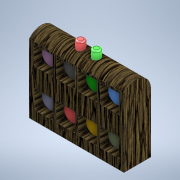
# Autodesk Inventor part: TreasureChestFinal
Saved by Autodesk Inventor 2021 (Build 250183000, 183)
## iProperties
Created: 2021-03-02
Part Number: TreasureChestFinal
Material: Generic
Document SubType Name: Modeling
Designer: con_c_000
Density: 1 g/cm^3
Appearance: Default
Author: con_c_000
Autodesk Inventor part; units mm, degrees
ref_plane "YZ Plane" through (0, 0, 0) normal (1, 0, 0) x (0, 1, 0)
ref_plane "XZ Plane" through (0, 0, 0) normal (0, 1, 0) x (-1, 0, 0)
ref_plane "XY Plane" through (0, 0, 0) normal (0, 0, 1) x (1, 0, 0)
sketch "Sketch1" plane through (0, 0, 0) normal (0, 1, 0) x (-1, 0, 0)
  line L0 (923.5659, 4.2179) -> (-600.4341, 4.2179)
  line L1 (-600.4341, 4.2179) -> (-600.4341, -300.5821)
  line L2 (-600.4341, -300.5821) -> (923.5659, -300.5821)
  line L3 (923.5659, -300.5821) -> (923.5659, 4.2179)
  point P0 (0, 0)
  dimension "d0" = 1524
  dimension "d1" = 304.8
  constraints: 8 end point, 2 parallel, 1 horizontal, 1 perpendicular
  measures "d0" distance of L2.end L1.end
  measures "d1" distance of L1.end L0.end
extrude "Extrusion1" add sketch "Sketch1" along normal blind 1219.2
sketch "Sketch2" plane through (-923.5659, 0, 4.2179) normal (0, 0, 1) x (1, 0, 0)
  circle A0 centre (228.6, 304.8) radius 127
  circle A1 centre (584.2, 304.8) radius 127
  circle A2 centre (939.8, 304.8) radius 127
  circle A3 centre (1295.4, 304.8) radius 127
  circle A4 centre (1295.4, 914.4) radius 127
  circle A5 centre (939.8, 914.4) radius 127
  circle A6 centre (584.2, 914.4) radius 127
  circle A7 centre (228.6, 914.4) radius 127
  line L0 (1524, 0) -> (1524, 1219.2) projected
  line L1 (0, 0) -> (0, 1219.2) projected
  line L2 (0, 1219.2) -> (1524, 1219.2) projected
  point P0 (923.5659, 0)
  dimension "d11" = 254
  dimension "d19" = 355.6
  dimension "d20" = 355.6
  dimension "d21" = 304.8
  dimension "d22" = 609.6
  dimension "d23" = 355.6
  dimension "d24" = 228.6
  constraints: 8 centre point, 7 equal radius, 6 horizontal alignment, 4 vertical alignment
  measures "d11" diameter of A7
  measures "d19" distance of A6.centre A5.centre
  measures "d20" distance of A4.centre A5.centre
  measures "d21" distance from line of L2 A7.centre
  measures "d22" distance of A0.centre A7.centre
  measures "d23" distance of A6.centre A7.centre
  measures "d24" distance from line of L1 A7.centre
extrude "Extrusion2" add sketch "Sketch2" along normal blind 25.4
sketch "Sketch3" plane through (-923.5659, 0, 4.2179) normal (0, 0, 1) x (1, 0, 0)
  line L0 (0, 1219.2) -> (1524, 1219.2) projected
  line L1 (0, 1219.2) -> (1524, 1219.2)
  line L2 (1524, 1219.2) -> (1524, 0)
  line L3 (1524, 0) -> (0, 0)
  line L4 (0, 0) -> (0, 1219.2)
  line L5 (76.2, 1066.8) -> (381, 1066.8)
  line L6 (381, 1066.8) -> (381, 762)
  line L7 (381, 762) -> (76.2, 762)
  line L8 (76.2, 762) -> (76.2, 1066.8)
  line L9 (431.8, 762) -> (736.6, 762)
  line L10 (736.6, 762) -> (736.6, 1066.8)
  line L11 (736.6, 1066.8) -> (431.8, 1066.8)
  line L12 (431.8, 1066.8) -> (431.8, 762)
  line L13 (787.4, 1066.8) -> (1092.2, 1066.8)
  line L14 (1092.2, 1066.8) -> (1092.2, 762)
  line L15 (1092.2, 762) -> (787.4, 762)
  line L16 (787.4, 762) -> (787.4, 1066.8)
  line L17 (1143, 762) -> (1447.8, 762)
  line L18 (1447.8, 762) -> (1447.8, 1066.8)
  line L19 (1447.8, 1066.8) -> (1143, 1066.8)
  line L20 (1143, 1066.8) -> (1143, 762)
  line L21 (84.918, 457.2) -> (381, 457.2)
  line L22 (381, 457.2) -> (381, 152.4)
  line L23 (381, 152.4) -> (84.918, 152.4)
  line L24 (84.918, 152.4) -> (84.918, 457.2)
  line L25 (431.8, 152.4) -> (736.6, 152.4)
  line L26 (736.6, 152.4) -> (736.6, 457.2)
  line L27 (736.6, 457.2) -> (431.8, 457.2)
  line L28 (431.8, 457.2) -> (431.8, 152.4)
  line L29 (787.4, 457.2) -> (1092.2, 457.2)
  line L30 (1092.2, 457.2) -> (1092.2, 152.4)
  line L31 (1092.2, 152.4) -> (787.4, 152.4)
  line L32 (787.4, 152.4) -> (787.4, 457.2)
  line L33 (1143, 152.4) -> (1447.8, 152.4)
  line L34 (1447.8, 152.4) -> (1447.8, 457.2)
  line L35 (1447.8, 457.2) -> (1143, 457.2)
  line L36 (1143, 457.2) -> (1143, 152.4)
  point P0 (923.5659, 0)
  point P1 (1524, 1219.2)
  dimension "d25" = 304.8
  dimension "d26" = 304.8
  dimension "d27" = 152.4
  dimension "d28" = 50.8
  dimension "d29" = 76.2
  dimension "d30" = 50.8
  dimension "d31" = 50.8
  dimension "d32" = 0
  dimension "d33" = 0
  dimension "d34" = 0
  dimension "d35" = 304.8
  dimension "d36" = 304.8
  dimension "d37" = 0
  constraints: 72 end point, 17 parallel, 13 point on line, 10 horizontal, 9 perpendicular, 5 equal length
  measures "d25" distance of L5.start L5.end
  measures "d26" distance of L7.end L5.start
  measures "d27" distance between parallel lines of L0 L5
  measures "d28" distance between parallel lines of L6 L12
  measures "d29" distance between parallel lines of L4 L8
  measures "d30" distance between parallel lines of L16 L10
  measures "d31" distance between parallel lines of L20 L14
  measures "d32" distance between parallel lines of L13 L19
  measures "d33" distance between parallel lines of L34 L18
  measures "d34" distance between parallel lines of L27 L21
  measures "d35" distance of L23.end L21.start
  measures "d36" distance between parallel lines of L7 L21
  measures "d37" distance between parallel lines of L25 L31
extrude "Extrusion3" add sketch "Sketch3" along normal blind 127
sketch "Sketch5" plane through (0, 1219.2, 0) normal (0, 1, 0) x (1, 0, 0)
  line L0 (600.4341, 300.5821) -> (600.4341, -131.2179) projected
  line L1 (600.4341, 300.5821) -> (-923.5659, 300.5821) projected
  line L2 (-923.5659, 300.5821) -> (-923.5659, -131.2179) projected
  line L3 (600.4341, -131.2179) -> (-923.5659, -131.2179) projected
  point P0 (0, 0)
extrude "Extrusion4" add sketch "Sketch5" along normal blind 254
sketch "Sketch6" plane through (-923.5659, 0, -300.5821) normal (-1, 0, 0) x (0, 0, 1)
  line L0 (431.8, 0) -> (431.8, 1473.2) projected
  line L1 (0, 0) -> (0, 1473.2) projected
  arc A0 (431.8, 1102.0767) -> (0, 944.9143) centre (239.7521, 957.9625) ccw
  line L2 (431.8, 1102.0767) -> (0, 944.9143) construction
  line L3 (431.8, 1102.0767) -> (891.312, 1102.0767) construction
  line L4 (0, 944.9143) -> (431.8, 944.9143)
  line L5 (431.8, 944.9143) -> (431.8, 1473.2)
  line L6 (431.8, 1473.2) -> (0, 1473.2)
  line L7 (0, 1473.2) -> (0, 944.9143)
  point P0 (300.5821, 0)
  point P1 (0, 971.0107)
  dimension "d42" = 160
  constraints: 12 end point, 2 horizontal, 2 parallel, 2 point on circle, 2 point on line, 1 centre point, 1 equal length, 1 perpendicular
  measures "d42" angle of L2 L3
extrude "Extrusion5" cut sketch "Sketch6" against normal through all contours A0 L1 L6 L0
ref_plane "Work Plane1" through (-923.5659, 1198.0694, -60.83) normal (0, -1, 0) x (1, 0, 0)
sketch "Sketch7" plane through (-923.5659, 1198.0694, -60.83) normal (0, -1, 0) x (1, 0, 0)
  circle A0 centre (635, 0.1041) radius 63.5
  circle A1 centre (889, 0.1041) radius 63.5
  line L0 (1524, -239.7521) -> (1524, 192.0479) projected
  line L1 (0, 192.0479) -> (0, -239.7521) projected
  point P0 (923.5659, 60.83)
  dimension "d45" = 127
  dimension "d46" = 127
  dimension "d47" = 635
  dimension "d48" = 635
  constraints: 2 centre point
  measures "d45" diameter of A0
  measures "d46" diameter of A1
  measures "d47" distance from line of L0 A1.centre
  measures "d48" distance from line of L1 A0.centre
extrude "Extrusion6" add sketch "Sketch7" along normal mid plane 254 from surface at 0
fillet "Fillet1" radius 25.4 2 edges at (-352.0659, 1325.0694, -60.7259) (-98.0659, 1325.0694, -60.7259)
equation "\"d19\" = d14"
equation "\"d20\" = d14"
equation "\"d22\" = 2 * d21"
equation "\"d23\" = d14"
equation "\"d30\" = d28"
equation "\"d31\" = d28"
equation "\"d14\" = 355.6"
body "Solid1"
